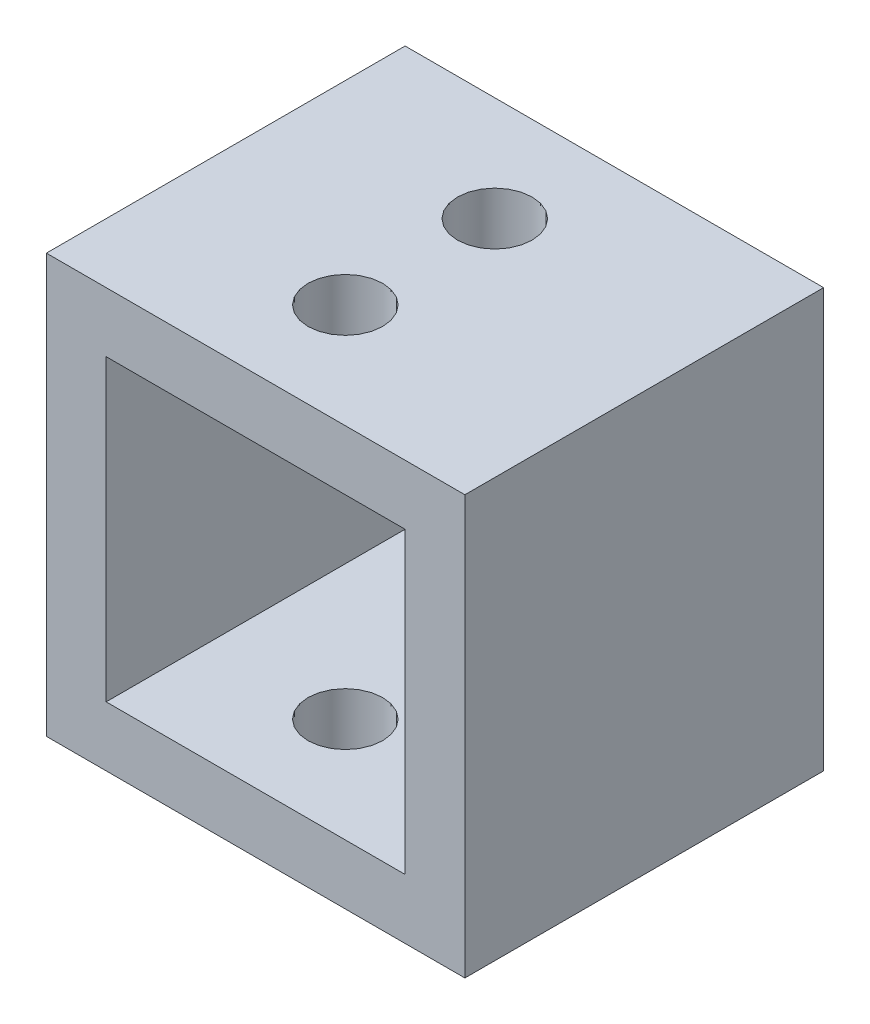
# Autodesk Inventor part: Aluminium2020-connector
Saved by Autodesk Inventor 2025 (Build 290162000, 162)
## iProperties
Created: 2024-05-24
Part Number: Aluminium2020-connector
Material: Generic
Document SubType Name: Modeling
Designer: hifzh
Density: 1 g/cm^3
Appearance: Default
Author: hifzh
Autodesk Inventor part; units mm, degrees
ref_plane "YZ Plane" through (0, 0, 0) normal (1, 0, 0) x (0, 1, 0)
ref_plane "XZ Plane" through (0, 0, 0) normal (0, 1, 0) x (-1, 0, 0)
ref_plane "XY Plane" through (0, 0, 0) normal (0, 0, 1) x (1, 0, 0)
sketch "Sketch1" plane through (0, 0, 0) normal (0, 0, 1) x (1, 0, 0)
  line L0 (0, 28) -> (28, 28)
  line L1 (28, 28) -> (28, 0)
  line L2 (28, 0) -> (0, 0)
  line L3 (0, 0) -> (0, 28)
  line L4 (4, 24) -> (24, 24)
  line L5 (24, 24) -> (24, 4)
  line L6 (24, 4) -> (4, 4)
  line L7 (4, 4) -> (4, 24)
  point P0 (14, 24)
  dimension "d1" = 28
  dimension "d3" = 20
  dimension "d4" = 4
  dimension "d5" = 4
  dimension "d6" = 28
  dimension "d7" = 20
  constraints: 16 end point, 4 perpendicular, 2 horizontal, 2 parallel, 1 midpoint
  measures "d1" distance of L0.end L1.end
  measures "d3" distance of L4.end L5.end
  measures "d4" distance between parallel lines of L7 L3
  measures "d5" distance from line of L0 point (14, 24)
  measures "d6" distance of L0.start L0.end
  measures "d7" distance of L4.start L4.end
sketch "Sketch2" plane through (0, 0, 0) normal (0, 1, 0) x (-1, 0, 0)
  line L0 (0, 0) -> (0, -24)
  line L1 (0, -24) -> (-26, -24)
  line L2 (-26, -24) -> (-26, 0)
  circle A0 centre (-13, -17) radius 2.5
  circle A1 centre (-13, -7) radius 2.5
  line L3 (-26, 0) -> (0, 0)
  dimension "d8" = 24
  dimension "d9" = 26
  dimension "d10" = 24
  dimension "d13" = 7
  dimension "d14" = 13
  dimension "d15" = 5
  dimension "d16" = 13
  dimension "d17" = 7
  dimension "d18" = 5
  constraints: 8 end point, 2 centre point, 2 perpendicular, 1 vertical
  measures "d8" distance of L0.start L0.end
  measures "d9" distance of L0.end L1.end
  measures "d10" distance of L1.end L2.end
  measures "d13" distance from line of A0.centre L1
  measures "d14" distance from line of L2 A0.centre
  measures "d15" diameter of A0
  measures "d16" distance from line of A1.centre L2
  measures "d17" distance from line of A1.centre L3
  measures "d18" diameter of A1
extrude "Extrusion1" add sketch "Sketch1" against normal blind 24
extrude "Extrusion2" cut sketch "Sketch2" along normal blind 29.975 contours A0 | A1
body "Solid1"
